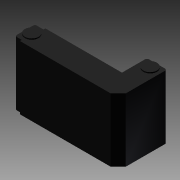
# Autodesk Inventor part: Bicep
Saved by Autodesk Inventor 2012 (Build 160160000, 160)
## iProperties
Created: 2013-02-21
Part Number: Bicep
Material: Default
Document SubType Name: Modeling
Designer: Andrew
Density: 1 g/cm^3
Author: Andrew
Autodesk Inventor part; units mm, degrees
ref_plane "YZ Plane" through (0, 0, 0) normal (1, 0, 0) x (0, 1, 0)
ref_plane "XZ Plane" through (0, 0, 0) normal (0, 1, 0) x (-1, 0, 0)
ref_plane "XY Plane" through (0, 0, 0) normal (0, 0, 1) x (1, 0, 0)
sketch "Sketch1" plane through (0, 0, 0) normal (0, 0, 1) x (1, 0, 0)
  arc A0 (-5.1284, 30.1824) -> (-4.7861, 30.3893) centre (0.7317, 20.8733) ccw
  circle A1 centre (0.7317, 20.8733) radius 11
  circle A2 centre (-141.2963, -27.3767) radius 11
  line L0 (-141.2963, -27.3767) -> (0.7317, -27.3767)
  line L1 (0.7317, -27.3767) -> (0.7317, 20.8733)
  line L2 (-70.2823, -27.3767) -> (-70.2823, -8.3767)
  line L3 (-70.2823, -27.3767) -> (-70.2823, -46.3767)
  line L4 (-141.2963, -11.3767) -> (-149.2963, -11.3767)
  line L5 (-152.2963, -14.3767) -> (-152.2963, -27.3767)
  line L6 (-152.2963, -27.3767) -> (-152.2963, -40.3767)
  line L7 (-141.2963, -11.3767) -> (-138.2963, -11.3767)
  line L8 (-138.2963, -11.3767) -> (-138.2963, -8.3767)
  line L9 (-138.2963, -8.3767) -> (-70.2823, -8.3767)
  line L10 (-141.2963, -46.3767) -> (-70.2823, -46.3767)
  line L11 (-12.2683, 31.8733) -> (13.7317, 31.8733)
  line L12 (4.7317, -46.3767) -> (-70.2823, -46.3767)
  line L13 (-15.2683, -8.3767) -> (-70.2823, -8.3767)
  line L14 (-141.2963, -46.3767) -> (-141.2963, -43.3767)
  line L15 (-141.2963, -43.3767) -> (-149.2963, -43.3767)
  line L16 (-15.2683, 20.8733) -> (-15.2683, -8.3767)
  line L17 (-15.2683, 20.8733) -> (-15.2683, 28.8733)
  line L18 (-12.2683, 31.8733) -> (-12.2683, 31.8733)
  line L19 (16.7317, 20.8733) -> (16.7317, 28.8733)
  line L20 (16.7317, 20.8733) -> (16.7317, -34.3767)
  line L21 (16.7317, -34.3767) -> (4.7317, -46.3767)
  arc A3 (-149.2963, -11.3767) -> (-152.2963, -14.3767) centre (-149.2963, -14.3767) ccw
  arc A4 (-152.2963, -40.3767) -> (-149.2963, -43.3767) centre (-149.2963, -40.3767) ccw
  arc A5 (-12.2683, 31.8733) -> (-15.2683, 28.8733) centre (-12.2683, 28.8733) ccw
  arc A6 (16.7317, 28.8733) -> (13.7317, 31.8733) centre (13.7317, 28.8733) ccw
  point P0 (16.7317, -46.3767)
  dimension "d8" = 22
  dimension "d9" = 19
  dimension "d10" = 16
  dimension "d12" = 19
  dimension "d15" = 3
  dimension "d17" = 16
  dimension "d18" = 16
  dimension "d19" = 12
  dimension "d20" = 12
  dimension "d21" = 3
  dimension "d22" = 3
  constraints: 44 end point, 8 point on circle, 8 tangent, 6 perpendicular, 5 centre point, 3 equal radius, 2 collinear, 2 vertical, 1 horizontal alignment, 1 midpoint, 1 parallel, 1 point on line, 2 other
  measures "d9" distance of L2.start L2.end
  measures "d10" distance of L0.start L4.start
  measures "d12" distance of L2.start L3.end
  measures "d15" distance of L4.start L7.end
  measures "d17" distance of L1.end L16.start
  measures "d18" distance of L1.end L19.start
  measures "d19" distance of L20.end point (16.732, -46.377)
  measures "d20" distance of L12.start point (16.732, -46.377)
  measures "d21" radius of A3
  measures "d22" radius of A5
extrude "Extrusion1" add sketch "Sketch1" along normal mid plane 102
extrude "Extrusion4" add sketch "Sketch1" along normal mid plane 105.5 contours A1 A0 | A2
equation "\"d20\" = d19"
body "Solid1"
